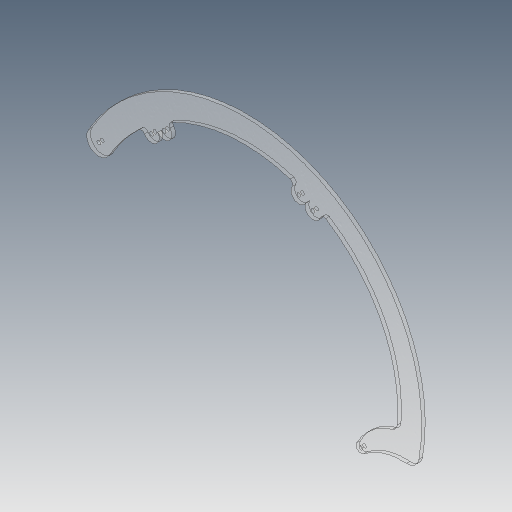
# Autodesk Inventor part: RailWay
Saved by Autodesk Inventor 2019.4 (Build 234330000, 330)
## iProperties
Created: 2019-06-11
Part Number: RailWay
Material: アクリル、クリア
Document SubType Name: Modeling
Designer: AzLIer
Density: 1.19 g/cm^3
Appearance: 透明 - クリア
Mass: 24.7622 g
Surface Area: 191.656 cm^2
Volume: 24.7622 cm^3
Author: AzLIer
Autodesk Inventor part; units mm, degrees
note: some values were not read from the file. Chosen so that the rebuilt part matches the saved one: sketch regions of "押し出し1".
ref_plane "YZ Plane" through (0, 0, 0) normal (1, 0, 0) x (0, 1, 0)
ref_plane "XZ Plane" through (0, 0, 0) normal (0, 1, 0) x (-1, 0, 0)
ref_plane "XY Plane" through (0, 0, 0) normal (0, 0, 1) x (1, 0, 0)
sketch "スケッチ1" plane through (0, 0, 0) normal (0, 0, 1) x (1, 0, 0)
  arc A0 (137.8731, -24.3107) -> (-121.2436, 70) centre (0, 0) ccw construction
  arc A1 (147.7212, -26.0472) -> (-129.9038, 75) centre (0, 0) ccw
  arc A2 (128.025, -22.5743) -> (-112.5833, 65) centre (0, 0) ccw
  arc A3 (128.025, -22.5743) -> (147.7212, -26.0472) centre (137.8731, -24.3107) ccw
  arc A4 (-129.9038, 75) -> (-112.5833, 65) centre (-121.2436, 70) ccw
  line L0 (0, 0) -> (0, 140) construction
  circle A5 centre (-121.2436, 70) radius 1.6
  circle A6 centre (98.9531, -42) radius 1.6
  arc A7 (95.4012, -40.1605) -> (101.4586, -45.1181) centre (98.9531, -42) ccw
  circle A8 centre (-76.9577, 98.5013) radius 1.6
  circle A9 centre (-66.2399, 106.006) radius 1.6
  circle A10 centre (0, 0) radius 125 construction
  arc A11 (-82.7322, 95.4269) -> (-87.3972, 96.2379) centre (-85.3803, 94.017) ccw
  arc A12 (-60.5425, 115.0418) -> (-61.3759, 110.3808) centre (-59.1453, 112.387) ccw
  arc A13 (-82.7322, 95.4269) -> (-71.5988, 102.2537) centre (-76.9577, 98.5013) ccw
  line L1 (-71.5988, 102.2537) -> (-74.5649, 106.4898)
  line L2 (-74.5649, 106.4898) -> (-71.5988, 102.2537)
  arc A14 (-71.5988, 102.2537) -> (-61.3759, 110.3808) centre (-66.2399, 106.006) ccw
  circle A15 centre (58.6839, 110.3684) radius 1.6
  arc A16 (69.3579, 109.9522) -> (64.9046, 108.3435) centre (67.7573, 107.4148) ccw
  arc A17 (52.7549, 113.1332) -> (64.9046, 108.3435) centre (58.6839, 110.3684) ccw
  circle A18 centre (46.8258, 115.898) radius 1.6
  line L3 (52.7549, 113.1332) -> (54.9404, 117.82)
  line L4 (54.9404, 117.82) -> (52.7549, 113.1332)
  arc A19 (41.276, 119.3617) -> (52.7549, 113.1332) centre (46.8258, 115.898) ccw
  arc A20 (41.276, 119.3617) -> (39.6459, 123.8071) centre (38.731, 120.95) ccw
  arc A21 (69.3579, 109.9522) -> (39.6459, 123.8071) centre (48.7491, 104.5427) ccw
  circle A22 centre (98.9531, -42) radius 1.6 projected
  arc A23 (137.0238, -34.2746) -> (101.4586, -45.1181) centre (132.7776, -84.094) ccw
  arc A24 (125.3649, -15.283) -> (95.4012, -40.1605) centre (139.8007, -63.1537) ccw
  arc A25 (125.3649, -15.283) -> (129.6148, -10) centre (123.6326, -9.5385) ccw
  dimension "d0" = 140
  dimension "d1" = 10
  dimension "d4" = 60
  dimension "d5" = 100
  dimension "d6" = 3.2
  dimension "d17" = 8
  dimension "d19" = 3.2
  dimension "d21" = 250
  dimension "d22" = 22
  dimension "d23" = 28
  dimension "d26" = 3
  dimension "d30" = 60
  dimension "d53" = 3.2
  dimension "d54" = 21.307
  dimension "d56" = 50
  dimension "d57" = 6
  dimension "d58" = 50
  dimension "d59" = 10
  constraints: 44 point on circle, 25 centre point, 14 tangent, 10 end point, 9 coincident, 3 equal radius, 2 line through centre, 1 collinear, 1 vertical, 22 other
  measures "d0" radius of A0
  measures "d1" radius of A3
  measures "d6" diameter of A5
  measures "d17" diameter of A7
  measures "d19" diameter of A8
  measures "d21" diameter of A10
  measures "d26" radius of A11
  measures "d53" diameter of A6
  measures "d54" radius of A21
  measures "d56" radius of A23
  measures "d57" radius of A25
  measures "d58" radius of A24
  measures "d59" vertical distance of point (0, 0) A25.end
extrude "押し出し1" add sketch "スケッチ1" along normal blind 3 contours A3 A2 A21 A4 A1 | A23 A7 A24 A25 A2 A3 | A2 L1 A13 A11 | A2 A12 A14 L1 | A2 A21 | A5
sketch "スケッチ3" plane through (0, 0, 0) normal (0, 0, 1) x (1, 0, 0)
  arc A0 (137.8731, -24.3107) -> (-121.2436, 70) centre (0, 0) ccw construction
  arc A1 (147.7212, -26.0472) -> (-129.9038, 75) centre (0, 0) ccw
  arc A2 (128.025, -22.5743) -> (147.7212, -26.0472) centre (137.8731, -24.3107) ccw
  arc A3 (-129.9038, 75) -> (-112.5833, 65) centre (-121.2436, 70) ccw
  line L0 (0, 0) -> (0, 140) construction
  circle A4 centre (-121.2436, 70) radius 1.6
  circle A5 centre (122.3274, -44) radius 1.6
  arc A6 (122.6106, -49.4927) -> (125.9627, -48.1273) centre (122.3274, -44) ccw
  line L1 (125.9627, -48.1273) -> (144.4827, -31.8149)
  circle A7 centre (102.9531, -46) radius 1.6
  arc A8 (102.4785, -41.5251) -> (103.1848, -50.494) centre (102.9531, -46) ccw
  line L2 (122.6106, -49.4927) -> (103.1848, -50.494)
  arc A9 (102.4785, -41.5251) -> (129.1083, -15.2002) centre (99.3141, -11.6925) ccw
  circle A10 centre (-76.9577, 98.5013) radius 1.6
  circle A11 centre (-66.2399, 106.006) radius 1.6
  circle A12 centre (0, 0) radius 125 construction
  arc A13 (-82.7322, 95.4269) -> (-87.3972, 96.2379) centre (-85.3803, 94.017) ccw
  arc A14 (-60.5425, 115.0418) -> (-61.3759, 110.3808) centre (-59.1453, 112.387) ccw
  arc A15 (-82.7322, 95.4269) -> (-71.5988, 102.2537) centre (-76.9577, 98.5013) ccw
  line L3 (-71.5988, 102.2537) -> (-74.5649, 106.4898)
  line L4 (-74.5649, 106.4898) -> (-71.5988, 102.2537)
  arc A16 (-71.5988, 102.2537) -> (-61.3759, 110.3808) centre (-66.2399, 106.006) ccw
  circle A17 centre (58.6839, 110.3684) radius 1.6
  arc A18 (69.3579, 109.9522) -> (64.9046, 108.3435) centre (67.7573, 107.4148) ccw
  arc A19 (52.7549, 113.1332) -> (64.9046, 108.3435) centre (58.6839, 110.3684) ccw
  circle A20 centre (46.8258, 115.898) radius 1.6
  line L5 (52.7549, 113.1332) -> (54.9404, 117.82)
  line L6 (54.9404, 117.82) -> (52.7549, 113.1332)
  arc A21 (41.276, 119.3617) -> (52.7549, 113.1332) centre (46.8258, 115.898) ccw
  arc A22 (41.276, 119.3617) -> (39.6459, 123.8071) centre (38.731, 120.95) ccw
  arc A23 (69.3579, 109.9522) -> (39.6459, 123.8071) centre (0, 0) ccw
  dimension "d34" = 140
  dimension "d35" = 10
  dimension "d36" = 60
  dimension "d37" = 100
  dimension "d38" = 3.2
  dimension "d39" = 11
  dimension "d40" = 9
  dimension "d41" = 30
  dimension "d42" = 3.2
  dimension "d43" = 250
  dimension "d44" = 22
  dimension "d45" = 28
  dimension "d46" = 3
  dimension "d47" = 60
  constraints: 37 point on circle, 24 centre point, 14 end point, 10 tangent, 9 coincident, 3 equal radius, 1 collinear, 1 vertical, 24 other
  measures "d34" radius of A0
  measures "d35" radius of A2
  measures "d38" diameter of A4
  measures "d39" diameter of A6
  measures "d40" diameter of A8
  measures "d41" radius of A9
  measures "d42" diameter of A10
  measures "d43" diameter of A12
  measures "d46" radius of A13
extrude "押し出し3" add sketch "スケッチ3" along normal blind 3 contours A18 A19 L5 A23 | L5 A21 A22 A23
sketch "スケッチ4" plane through (0, 0, 3) normal (0, 0, 1) x (1, 0, 0)
  circle A0 centre (58.6839, 110.3684) radius 1.6 projected
  circle A1 centre (46.8258, 115.898) radius 1.6 projected
  circle A2 centre (98.9531, -42) radius 1.6 projected
  arc A3 (125.3649, -15.283) -> (129.6148, -10) centre (123.6326, -9.5385) ccw projected
  arc A4 (125.3649, -15.283) -> (95.4012, -40.1605) centre (139.8007, -63.1537) ccw projected
  arc A5 (95.4012, -40.1605) -> (101.4586, -45.1181) centre (98.9531, -42) ccw projected
  arc A6 (137.0238, -34.2746) -> (101.4586, -45.1181) centre (132.7776, -84.094) ccw projected
  arc A7 (137.0238, -34.2746) -> (147.7212, -26.0472) centre (137.8731, -24.3107) ccw projected
  arc A8 (147.7212, -26.0472) -> (-129.9038, 75) centre (0, 0) ccw projected
  arc A9 (-129.9038, 75) -> (-112.5833, 65) centre (-121.2436, 70) ccw projected
  arc A10 (-87.3972, 96.2379) -> (-112.5833, 65) centre (0, 0) ccw projected
  arc A11 (-82.7322, 95.4269) -> (-87.3972, 96.2379) centre (-85.3803, 94.017) ccw projected
  arc A12 (-82.7322, 95.4269) -> (-71.5988, 102.2537) centre (-76.9577, 98.5013) ccw projected
  arc A13 (-71.5988, 102.2537) -> (-61.3759, 110.3808) centre (-66.2399, 106.006) ccw projected
  arc A14 (-60.5425, 115.0418) -> (-61.3759, 110.3808) centre (-59.1453, 112.387) ccw projected
  arc A15 (39.6459, 123.8071) -> (-60.5425, 115.0418) centre (0, 0) ccw projected
  arc A16 (41.276, 119.3617) -> (39.6459, 123.8071) centre (38.731, 120.95) ccw projected
  arc A17 (41.276, 119.3617) -> (52.7549, 113.1332) centre (46.8258, 115.898) ccw projected
  arc A18 (52.7549, 113.1332) -> (64.9046, 108.3435) centre (58.6839, 110.3684) ccw projected
  arc A19 (69.3579, 109.9522) -> (64.9046, 108.3435) centre (67.7573, 107.4148) ccw projected
  arc A20 (129.6148, -10) -> (69.3579, 109.9522) centre (0, 0) ccw projected
  circle A21 centre (-66.2399, 106.006) radius 1.6 projected
  circle A22 centre (-76.9577, 98.5013) radius 1.6 projected
  circle A23 centre (-121.2436, 70) radius 1.6
  dimension "d60" = 3.2
  constraints: 1 centre point, 1 coincident
  measures "d60" diameter of A23
extrude "押し出し4" cut sketch "スケッチ4" against normal blind 10 contours A23
